Autodesk Inventor part; units mm, degrees
(part 2 of 2)
sketch "Sketch4" plane through (-0.0003, -144.9621, 0) normal (0, -1, 0) x (-0.0016, 0, -1)
  line L0 (16.9376, 64.7399) -> (58.7136, 64.7399) construction
  line L1 (58.7136, 64.7399) -> (58.7136, 48.1903) construction
  line L2 (58.7136, 48.1903) -> (16.9376, 48.1903) construction
  line L3 (16.9376, 48.1903) -> (16.9376, 64.7399) construction
  line L4 (19.529, 58.6329) -> (17.2049, 58.6329)
  line L5 (17.2049, 58.6329) -> (17.2049, 59.2456)
  line L6 (17.2049, 59.2456) -> (17.9682, 59.2456)
  line L7 (17.9682, 59.2456) -> (17.9682, 64.0203)
  line L8 (17.9682, 64.0203) -> (17.2049, 64.0203)
  line L9 (17.2049, 64.0203) -> (17.2049, 64.6329)
  line L10 (17.2049, 64.6329) -> (19.529, 64.6329)
  line L11 (19.529, 64.6329) -> (19.529, 64.0203)
  line L12 (19.529, 64.0203) -> (18.7656, 64.0203)
  line L13 (18.7656, 64.0203) -> (18.7656, 59.2456)
  line L14 (18.7656, 59.2456) -> (19.529, 59.2456)
  line L15 (19.529, 59.2456) -> (19.529, 58.6329)
  line L16 (24.8094, 58.6329) -> (23.9148, 58.6329)
  line L17 (23.9148, 58.6329) -> (21.26, 63.8063)
  line L18 (21.26, 63.8063) -> (21.26, 58.6329)
  line L19 (21.26, 58.6329) -> (20.5161, 58.6329)
  line L20 (20.5161, 58.6329) -> (20.5161, 64.6329)
  line L21 (20.5161, 64.6329) -> (21.649, 64.6329)
  line L22 (21.649, 64.6329) -> (24.0655, 59.8825)
  line L23 (24.0655, 59.8825) -> (24.0655, 64.6329)
  line L24 (24.0655, 64.6329) -> (24.8094, 64.6329)
  line L25 (24.8094, 64.6329) -> (24.8094, 58.6329)
  line L26 (27.4253, 58.6329) -> (27.4253, 63.923)
  line L27 (27.4253, 63.923) -> (25.4123, 63.923)
  line L28 (25.4123, 63.923) -> (25.4123, 64.6329)
  line L29 (25.4123, 64.6329) -> (30.2357, 64.6329)
  line L30 (30.2357, 64.6329) -> (30.2357, 63.923)
  line L31 (30.2357, 63.923) -> (28.2227, 63.923)
  line L32 (28.2227, 63.923) -> (28.2227, 58.6329)
  line L33 (28.2227, 58.6329) -> (27.4253, 58.6329)
  line L34 (30.8434, 58.6329) -> (30.8434, 64.6329)
  line L35 (30.8434, 64.6329) -> (34.5971, 64.6329)
  line L36 (34.5971, 64.6329) -> (34.5971, 63.923)
  line L37 (34.5971, 63.923) -> (31.6409, 63.923)
  line L38 (31.6409, 63.923) -> (31.6409, 62.2796)
  line L39 (31.6409, 62.2796) -> (34.3977, 62.2796)
  line L40 (34.3977, 62.2796) -> (34.3977, 61.5697)
  line L41 (34.3977, 61.5697) -> (31.6409, 61.5697)
  line L42 (31.6409, 61.5697) -> (31.6409, 59.3428)
  line L43 (31.6409, 59.3428) -> (34.5971, 59.3428)
  line L44 (34.5971, 59.3428) -> (34.5971, 58.6329)
  line L45 (34.5971, 58.6329) -> (30.8434, 58.6329)
  line L46 (40.1157, 58.6329) -> (39.0801, 58.6329)
  line L47 (39.0801, 58.6329) -> (37.1838, 61.0203)
  line L48 (37.1838, 61.0203) -> (36.2697, 61.0203)
  line L49 (36.2697, 61.0203) -> (36.2697, 58.6329)
  line L50 (36.2697, 58.6329) -> (35.4723, 58.6329)
  line L51 (35.4723, 58.6329) -> (35.4723, 64.6329)
  line L52 (35.4723, 64.6329) -> (37.0185, 64.6329)
  spline S0 degree 2 poles (37.0185, 64.6329) (37.5339, 64.6329) (38.2292, 64.5211) (38.5452, 64.3169) knots 0 0 0 1 2 2 2
  spline S1 degree 2 poles (38.5452, 64.3169) (38.8613, 64.1127) (39.2259, 63.4757) (39.2259, 63.0041) knots 0 0 0 1 2 2 2
  spline S2 degree 2 poles (39.2259, 63.0041) (39.2259, 62.3477) (38.555, 61.4579) (37.9812, 61.2439) knots 0 0 0 1 2 2 2
  line L53 (37.9812, 61.2439) -> (40.1157, 58.6329)
  spline S3 degree 2 poles (38.3945, 62.9409) (38.3945, 63.2034) (38.2097, 63.607) (38.0152, 63.7383) knots 0 0 0 1 2 2 2
  spline S4 degree 2 poles (38.0152, 63.7383) (37.8451, 63.8501) (37.3929, 63.9425) (37.0622, 63.9425) knots 0 0 0 1 2 2 2
  line L54 (37.0622, 63.9425) -> (36.2697, 63.9425)
  line L55 (36.2697, 63.9425) -> (36.2697, 61.6864)
  line L56 (36.2697, 61.6864) -> (36.9699, 61.6864)
  spline S5 degree 2 poles (36.9699, 61.6864) (37.3151, 61.6864) (37.8645, 61.808) (38.0541, 61.9976) knots 0 0 0 1 2 2 2
  spline S6 degree 2 poles (38.0541, 61.9976) (38.2292, 62.1629) (38.3945, 62.6297) (38.3945, 62.9409) knots 0 0 0 1 2 2 2
  line L57 (44.1806, 63.923) -> (41.3896, 63.923)
  line L58 (41.3896, 63.923) -> (41.3896, 62.231)
  line L59 (41.3896, 62.231) -> (44.0639, 62.231)
  line L60 (44.0639, 62.231) -> (44.0639, 61.5211)
  line L61 (44.0639, 61.5211) -> (41.3896, 61.5211)
  line L62 (41.3896, 61.5211) -> (41.3896, 58.6329)
  line L63 (41.3896, 58.6329) -> (40.5922, 58.6329)
  line L64 (40.5922, 58.6329) -> (40.5922, 64.6329)
  line L65 (40.5922, 64.6329) -> (44.1806, 64.6329)
  line L66 (44.1806, 64.6329) -> (44.1806, 63.923)
  line L67 (44.2486, 58.6329) -> (46.2713, 64.6329)
  line L68 (46.2713, 64.6329) -> (47.2535, 64.6329)
  line L69 (47.2535, 64.6329) -> (49.2762, 58.6329)
  line L70 (49.2762, 58.6329) -> (48.435, 58.6329)
  line L71 (48.435, 58.6329) -> (47.8904, 60.3104)
  line L72 (47.8904, 60.3104) -> (45.6003, 60.3104)
  line L73 (45.6003, 60.3104) -> (45.0558, 58.6329)
  line L74 (45.0558, 58.6329) -> (44.2486, 58.6329)
  line L75 (47.6716, 60.9911) -> (46.743, 63.8161)
  line L76 (46.743, 63.8161) -> (45.8191, 60.9911)
  line L77 (45.8191, 60.9911) -> (47.6716, 60.9911)
  spline S7 degree 2 poles (52.1887, 58.5259) (51.6052, 58.5259) (50.6182, 58.9198) (50.2584, 59.3136) knots 0 0 0 1 2 2 2
  spline S8 degree 2 poles (50.2584, 59.3136) (49.8986, 59.7026) (49.5047, 60.8695) (49.5047, 61.6281) knots 0 0 0 1 2 2 2
  spline S9 degree 2 poles (49.5047, 61.6281) (49.5047, 62.3817) (49.8888, 63.5) (50.2535, 63.9133) knots 0 0 0 1 2 2 2
  spline S10 degree 2 poles (50.2535, 63.9133) (50.6133, 64.3169) (51.5955, 64.7399) (52.2033, 64.7399) knots 0 0 0 1 2 2 2
  spline S11 degree 2 poles (52.2033, 64.7399) (52.5047, 64.7399) (53.0347, 64.6524) (53.2584, 64.5843) knots 0 0 0 1 2 2 2
  spline S12 degree 2 poles (53.2584, 64.5843) (53.4528, 64.5211) (53.8564, 64.3412) (54.0558, 64.2342) knots 0 0 0 1 2 2 2
  line L78 (54.0558, 64.2342) -> (54.0558, 63.2715)
  line L79 (54.0558, 63.2715) -> (53.9926, 63.2715)
  spline S13 degree 2 poles (53.9926, 63.2715) (53.8856, 63.3687) (53.555, 63.641) (53.3167, 63.7723) knots 0 0 0 1 2 2 2
  spline S14 degree 2 poles (53.3167, 63.7723) (53.0882, 63.8987) (52.5485, 64.0592) (52.1984, 64.0592) knots 0 0 0 1 2 2 2
  spline S15 degree 2 poles (52.1984, 64.0592) (51.8143, 64.0592) (51.1287, 63.7431) (50.871, 63.4417) knots 0 0 0 1 2 2 2
  spline S16 degree 2 poles (50.871, 63.4417) (50.6182, 63.1353) (50.3362, 62.2067) (50.3362, 61.6281) knots 0 0 0 1 2 2 2
  spline S17 degree 2 poles (50.3362, 61.6281) (50.3362, 61.0106) (50.6327, 60.1208) (50.8904, 59.8144) knots 0 0 0 1 2 2 2
  spline S18 degree 2 poles (50.8904, 59.8144) (51.1433, 59.5178) (51.8191, 59.2164) (52.1984, 59.2164) knots 0 0 0 1 2 2 2
  spline S19 degree 2 poles (52.1984, 59.2164) (52.5436, 59.2164) (53.1319, 59.3866) (53.3605, 59.513) knots 0 0 0 1 2 2 2
  spline S20 degree 2 poles (53.3605, 59.513) (53.5793, 59.6394) (53.905, 59.902) (53.9974, 59.9943) knots 0 0 0 1 2 2 2
  line L80 (53.9974, 59.9943) -> (54.0558, 59.9943)
  line L81 (54.0558, 59.9943) -> (54.0558, 59.0413)
  spline S21 degree 2 poles (54.0558, 59.0413) (53.8564, 58.949) (53.5063, 58.7788) (53.2584, 58.701) knots 0 0 0 1 2 2 2
  spline S22 degree 2 poles (53.2584, 58.701) (52.9958, 58.6135) (52.5485, 58.5259) (52.1887, 58.5259) knots 0 0 0 1 2 2 2
  line L82 (54.7997, 58.6329) -> (54.7997, 64.6329)
  line L83 (54.7997, 64.6329) -> (58.5533, 64.6329)
  line L84 (58.5533, 64.6329) -> (58.5533, 63.923)
  line L85 (58.5533, 63.923) -> (55.5971, 63.923)
  line L86 (55.5971, 63.923) -> (55.5971, 62.2796)
  line L87 (55.5971, 62.2796) -> (58.354, 62.2796)
  line L88 (58.354, 62.2796) -> (58.354, 61.5697)
  line L89 (58.354, 61.5697) -> (55.5971, 61.5697)
  line L90 (55.5971, 61.5697) -> (55.5971, 59.3428)
  line L91 (55.5971, 59.3428) -> (58.5533, 59.3428)
  line L92 (58.5533, 59.3428) -> (58.5533, 58.6329)
  line L93 (58.5533, 58.6329) -> (54.7997, 58.6329)
  line L94 (27.6076, 48.7541) -> (26.8102, 48.7541)
  line L95 (26.8102, 48.7541) -> (26.8102, 53.9226)
  line L96 (26.8102, 53.9226) -> (25.2446, 50.4072)
  line L97 (25.2446, 50.4072) -> (24.7584, 50.4072)
  line L98 (24.7584, 50.4072) -> (23.2073, 53.9226)
  line L99 (23.2073, 53.9226) -> (23.2073, 48.7541)
  line L100 (23.2073, 48.7541) -> (22.4634, 48.7541)
  line L101 (22.4634, 48.7541) -> (22.4634, 54.7541)
  line L102 (22.4634, 54.7541) -> (23.5525, 54.7541)
  line L103 (23.5525, 54.7541) -> (25.0501, 51.4137)
  line L104 (25.0501, 51.4137) -> (26.499, 54.7541)
  line L105 (26.499, 54.7541) -> (27.6076, 54.7541)
  line L106 (27.6076, 54.7541) -> (27.6076, 48.7541)
  spline S23 degree 2 poles (33.0679, 54.0685) (33.4083, 53.6698) (33.7875, 52.5029) (33.7875, 51.7541) knots 0 0 0 1 2 2 2
  spline S24 degree 2 poles (33.7875, 51.7541) (33.7875, 51.0247) (33.418, 49.8432) (33.0679, 49.4445) knots 0 0 0 1 2 2 2
  spline S25 degree 2 poles (33.0679, 49.4445) (32.6984, 49.0264) (31.7211, 48.6277) (31.1327, 48.6277) knots 0 0 0 1 2 2 2
  spline S26 degree 2 poles (31.1327, 48.6277) (30.525, 48.6277) (29.5525, 49.0409) (29.1976, 49.4445) knots 0 0 0 1 2 2 2
  spline S27 degree 2 poles (29.1976, 49.4445) (28.8524, 49.8432) (28.4828, 51.015) (28.4828, 51.7541) knots 0 0 0 1 2 2 2
  spline S28 degree 2 poles (28.4828, 51.7541) (28.4828, 52.5077) (28.8572, 53.6552) (29.2024, 54.0685) knots 0 0 0 1 2 2 2
  spline S29 degree 2 poles (29.2024, 54.0685) (29.5525, 54.4672) (30.5298, 54.8805) (31.1327, 54.8805) knots 0 0 0 1 2 2 2
  spline S30 degree 2 poles (31.1327, 54.8805) (31.7454, 54.8805) (32.7276, 54.4526) (33.0679, 54.0685) knots 0 0 0 1 2 2 2
  spline S31 degree 2 poles (32.9561, 51.7541) (32.9561, 52.3473) (32.6984, 53.2662) (32.465, 53.5677) knots 0 0 0 1 2 2 2
  spline S32 degree 2 poles (32.465, 53.5677) (32.2268, 53.8789) (31.5558, 54.1901) (31.1376, 54.1901) knots 0 0 0 1 2 2 2
  spline S33 degree 2 poles (31.1376, 54.1901) (30.7049, 54.1901) (30.0533, 53.8886) (29.8054, 53.5677) knots 0 0 0 1 2 2 2
  spline S34 degree 2 poles (29.8054, 53.5677) (29.5671, 53.2614) (29.3143, 52.3375) (29.3143, 51.7541) knots 0 0 0 1 2 2 2
  spline S35 degree 2 poles (29.3143, 51.7541) (29.3143, 50.5726) (30.3062, 49.3181) (31.1376, 49.3181) knots 0 0 0 1 2 2 2
  spline S36 degree 2 poles (31.1376, 49.3181) (31.9691, 49.3181) (32.9561, 50.5726) (32.9561, 51.7541) knots 0 0 0 1 2 2 2
  spline S37 degree 2 poles (39.3937, 51.7492) (39.3937, 50.9275) (38.7276, 49.605) (38.1684, 49.2354) knots 0 0 0 1 2 2 2
  spline S38 degree 2 poles (38.1684, 49.2354) (37.7114, 48.9486) (36.7729, 48.7541) (36.0436, 48.7541) knots 0 0 0 1 2 2 2
  line L107 (36.0436, 48.7541) -> (34.6627, 48.7541)
  line L108 (34.6627, 48.7541) -> (34.6627, 54.7541)
  line L109 (34.6627, 54.7541) -> (36.029, 54.7541)
  spline S39 degree 2 poles (36.029, 54.7541) (36.8751, 54.7541) (37.8378, 54.5012) (38.1781, 54.2776) knots 0 0 0 1 2 2 2
  spline S40 degree 2 poles (38.1781, 54.2776) (38.7567, 53.8935) (39.3937, 52.6244) (39.3937, 51.7492) knots 0 0 0 1 2 2 2
  spline S41 degree 2 poles (38.5622, 51.7589) (38.5622, 52.4494) (38.1052, 53.4267) (37.653, 53.7038) knots 0 0 0 1 2 2 2
  spline S42 degree 2 poles (37.653, 53.7038) (37.3321, 53.8935) (36.6076, 54.0636) (36.0679, 54.0636) knots 0 0 0 1 2 2 2
  line L110 (36.0679, 54.0636) -> (35.4601, 54.0636)
  line L111 (35.4601, 54.0636) -> (35.4601, 49.4445)
  line L112 (35.4601, 49.4445) -> (36.0679, 49.4445)
  spline S43 degree 2 poles (36.0679, 49.4445) (36.5979, 49.4445) (37.4002, 49.6147) (37.7259, 49.8432) knots 0 0 0 1 2 2 2
  spline S44 degree 2 poles (37.7259, 49.8432) (38.1441, 50.1252) (38.5622, 51.0588) (38.5622, 51.7589) knots 0 0 0 1 2 2 2
  spline S45 degree 2 poles (42.3548, 48.6277) (41.8248, 48.6277) (41.0371, 48.9048) (40.76, 49.182) knots 0 0 0 1 2 2 2
  spline S46 degree 2 poles (40.76, 49.182) (40.4439, 49.4931) (40.1862, 50.3683) (40.1862, 51.0102) knots 0 0 0 1 2 2 2
  line L113 (40.1862, 51.0102) -> (40.1862, 54.7541)
  line L114 (40.1862, 54.7541) -> (40.9836, 54.7541)
  line L115 (40.9836, 54.7541) -> (40.9836, 51.0102)
  spline S47 degree 2 poles (40.9836, 51.0102) (40.9836, 50.592) (41.0906, 50.028) (41.2413, 49.7995) knots 0 0 0 1 2 2 2
  spline S48 degree 2 poles (41.2413, 49.7995) (41.4018, 49.5563) (41.9561, 49.3084) (42.3548, 49.3084) knots 0 0 0 1 2 2 2
  spline S49 degree 2 poles (42.3548, 49.3084) (42.7292, 49.3084) (43.3127, 49.5563) (43.4731, 49.7995) knots 0 0 0 1 2 2 2
  spline S50 degree 2 poles (43.4731, 49.7995) (43.6238, 50.028) (43.7308, 50.5871) (43.7308, 50.9907) knots 0 0 0 1 2 2 2
  line L116 (43.7308, 50.9907) -> (43.7308, 54.7541)
  line L117 (43.7308, 54.7541) -> (44.5282, 54.7541)
  line L118 (44.5282, 54.7541) -> (44.5282, 51.0102)
  spline S51 degree 2 poles (44.5282, 51.0102) (44.5282, 50.3829) (44.2754, 49.4883) (43.9545, 49.182) knots 0 0 0 1 2 2 2
  spline S52 degree 2 poles (43.9545, 49.182) (43.6676, 48.8999) (42.9091, 48.6277) (42.3548, 48.6277) knots 0 0 0 1 2 2 2
  line L119 (49.1473, 48.7541) -> (45.6708, 48.7541)
  line L120 (45.6708, 48.7541) -> (45.6708, 54.7541)
  line L121 (45.6708, 54.7541) -> (46.4682, 54.7541)
  line L122 (46.4682, 54.7541) -> (46.4682, 49.464)
  line L123 (46.4682, 49.464) -> (49.1473, 49.464)
  line L124 (49.1473, 49.464) -> (49.1473, 48.7541)
  line L125 (49.7746, 48.7541) -> (49.7746, 54.7541)
  line L126 (49.7746, 54.7541) -> (53.5282, 54.7541)
  line L127 (53.5282, 54.7541) -> (53.5282, 54.0442)
  line L128 (53.5282, 54.0442) -> (50.572, 54.0442)
  line L129 (50.572, 54.0442) -> (50.572, 52.4008)
  line L130 (50.572, 52.4008) -> (53.3289, 52.4008)
  line L131 (53.3289, 52.4008) -> (53.3289, 51.6909)
  line L132 (53.3289, 51.6909) -> (50.572, 51.6909)
  line L133 (50.572, 51.6909) -> (50.572, 49.464)
  line L134 (50.572, 49.464) -> (53.5282, 49.464)
  line L135 (53.5282, 49.464) -> (53.5282, 48.7541)
  line L136 (53.5282, 48.7541) -> (49.7746, 48.7541)
  point P0 (0, 0)
  constraints: 2 other
extrude "Extrusion4" add sketch "Sketch4" against normal blind 2
ref_plane "Work Plane5" through (-0.0003, -144.9621, -142.4319) normal (0, 0, -1) x (-1, 0, 0)
sketch "Sketch5" plane through (-0.0003, -144.9621, -142.4319) normal (0, 0, -1) x (-1, 0, 0)
  circle A0 centre (-58.0001, 28.9999) radius 17.5
  circle A1 centre (-58.0002, 115.962) radius 17.5
  spline S0 degree 2 poles (-56.1337, 59.9308) (-56.1337, 60.7898) (-55.9473, 61.9487) (-55.6069, 62.4754) knots -2 -2 -2 -1 0 0 0 projected
  spline S1 degree 2 poles (-55.6069, 62.4754) (-55.2666, 63.0022) (-54.205, 63.6099) (-53.4189, 63.6099) knots -2 -2 -2 -1 0 0 0 projected
  spline S2 degree 2 poles (-53.4189, 63.6099) (-52.3249, 63.6099) (-50.8419, 62.4916) (-50.4854, 61.5354) knots -2 -2 -2 -1 0 0 0 projected
  line L0 (-50.4854, 61.5354) -> (-46.1337, 65.0929) projected
  line L1 (-46.1337, 65.0929) -> (-46.1337, 63.3668) projected
  line L2 (-46.1337, 63.3668) -> (-50.1126, 60.2064) projected
  line L3 (-50.1126, 60.2064) -> (-50.1126, 58.6829) projected
  line L4 (-50.1126, 58.6829) -> (-46.1337, 58.6829) projected
  line L5 (-46.1337, 58.6829) -> (-46.1337, 57.3539) projected
  line L6 (-46.1337, 57.3539) -> (-56.1337, 57.3539) projected
  line L7 (-56.1337, 57.3539) -> (-56.1337, 59.9308) projected
  spline S3 degree 2 poles (-35.1604, 55.2567) (-35.692, 54.7964) (-37.2544, 54.3037) (-38.2398, 54.3037) knots -2 -2 -2 -1 0 0 0 projected
  spline S4 degree 2 poles (-38.2398, 54.3037) (-39.2446, 54.3037) (-40.7746, 54.8028) (-41.3257, 55.2631) knots -2 -2 -2 -1 0 0 0 projected
  spline S5 degree 2 poles (-41.3257, 55.2631) (-41.8573, 55.7299) (-42.4083, 57.033) (-42.4083, 57.8369) knots -2 -2 -2 -1 0 0 0 projected
  spline S6 degree 2 poles (-42.4083, 57.8369) (-42.4083, 58.6537) (-41.8378, 59.9633) (-41.3257, 60.4171) knots -2 -2 -2 -1 0 0 0 projected
  spline S7 degree 2 poles (-41.3257, 60.4171) (-40.7941, 60.8709) (-39.2382, 61.3766) (-38.2398, 61.3766) knots -2 -2 -2 -1 0 0 0 projected
  spline S8 degree 2 poles (-38.2398, 61.3766) (-37.2673, 61.3766) (-35.692, 60.8839) (-35.1604, 60.4171) knots -2 -2 -2 -1 0 0 0 projected
  spline S9 degree 2 poles (-35.1604, 60.4171) (-34.6028, 59.9244) (-34.0712, 58.6213) (-34.0712, 57.8369) knots -2 -2 -2 -1 0 0 0 projected
  spline S10 degree 2 poles (-34.0712, 57.8369) (-34.0712, 57.0265) (-34.6223, 55.7299) (-35.1604, 55.2567) knots -2 -2 -2 -1 0 0 0 projected
  line L8 (-38.1555, 82.7186) -> (-35.1863, 82.7186) projected
  line L9 (-35.1863, 82.7186) -> (-35.1863, 86.6602) projected
  line L10 (-35.1863, 86.6602) -> (-34.2398, 86.6602) projected
  line L11 (-34.2398, 86.6602) -> (-34.2398, 81.6554) projected
  line L12 (-34.2398, 81.6554) -> (-42.2398, 81.6554) projected
  line L13 (-42.2398, 81.6554) -> (-42.2398, 86.6602) projected
  line L14 (-42.2398, 86.6602) -> (-41.2933, 86.6602) projected
  line L15 (-41.2933, 86.6602) -> (-41.2933, 82.7186) projected
  line L16 (-41.2933, 82.7186) -> (-39.102, 82.7186) projected
  line L17 (-39.102, 82.7186) -> (-39.102, 86.3944) projected
  line L18 (-39.102, 86.3944) -> (-38.1555, 86.3944) projected
  line L19 (-38.1555, 86.3944) -> (-38.1555, 82.7186) projected
  line L20 (-42.2398, 76.1837) -> (-42.2398, 77.2469) projected
  line L21 (-42.2398, 77.2469) -> (-35.1863, 77.2469) projected
  line L22 (-35.1863, 77.2469) -> (-35.1863, 80.8191) projected
  line L23 (-35.1863, 80.8191) -> (-34.2398, 80.8191) projected
  line L24 (-34.2398, 80.8191) -> (-34.2398, 76.1837) projected
  line L25 (-34.2398, 76.1837) -> (-42.2398, 76.1837) projected
  line L26 (-16.862, 12.0764) -> (-28.862, 12.0764) projected
  line L27 (-28.862, 12.0764) -> (-28.862, 15.091) projected
  spline S11 degree 2 poles (-28.862, 15.091) (-28.862, 16.1607) (-28.5119, 17.6583) (-28.1132, 18.232) knots -2 -2 -2 -1 0 0 0 projected
  spline S12 degree 2 poles (-28.1132, 18.232) (-27.6561, 18.903) (-26.2461, 19.6615) (-25.2445, 19.6615) knots -2 -2 -2 -1 0 0 0 projected
  spline S13 degree 2 poles (-25.2445, 19.6615) (-24.4665, 19.6615) (-23.0662, 19.1072) (-22.58, 18.6113) knots -2 -2 -2 -1 0 0 0 projected
  spline S14 degree 2 poles (-22.58, 18.6113) (-21.9673, 17.9889) (-21.3352, 16.3066) (-21.3352, 15.0229) knots -2 -2 -2 -1 0 0 0 projected
  line L28 (-21.3352, 15.0229) -> (-21.3352, 13.6712) projected
  line L29 (-21.3352, 13.6712) -> (-16.862, 13.6712) projected
  line L30 (-16.862, 13.6712) -> (-16.862, 12.0764) projected
  line L31 (-10.1757, 135.4385) -> (-10.1757, 136.2683) projected
  line L32 (-10.1757, 136.2683) -> (-2.9666, 136.2683) projected
  line L33 (-2.9666, 136.2683) -> (-2.9666, 137.688) projected
  line L34 (-2.9666, 137.688) -> (-2.1497, 137.688) projected
  line L35 (-2.1497, 137.688) -> (-2.1497, 133.7853) projected
  line L36 (-2.1497, 133.7853) -> (-2.9666, 133.7853) projected
  line L37 (-2.9666, 133.7853) -> (-2.9666, 135.2375) projected
  line L38 (-2.9666, 135.2375) -> (-8.328, 135.2375) projected
  line L39 (-8.328, 135.2375) -> (-8.328, 133.7853) projected
  line L40 (-8.328, 133.7853) -> (-9.0606, 133.7853) projected
  spline S15 degree 2 poles (-9.0606, 133.7853) (-9.0606, 134.6086) (-9.5274, 135.3866) (-10.1757, 135.4385) knots -2 -2 -2 -1 0 0 0 projected
  line L41 (-46.0033, 83.678) -> (-46.0033, 82.349) projected
  line L42 (-46.0033, 82.349) -> (-56.0033, 82.349) projected
  line L43 (-56.0033, 82.349) -> (-56.0033, 88.3295) projected
  line L44 (-56.0033, 88.3295) -> (-54.8201, 88.3295) projected
  line L45 (-54.8201, 88.3295) -> (-54.8201, 83.678) projected
  line L46 (-54.8201, 83.678) -> (-52, 83.678) projected
  line L47 (-52, 83.678) -> (-52, 88.135) projected
  line L48 (-52, 88.135) -> (-50.8169, 88.135) projected
  line L49 (-50.8169, 88.135) -> (-50.8169, 83.678) projected
  line L50 (-50.8169, 83.678) -> (-46.0033, 83.678) projected
  line L51 (-42.2398, 67.1724) -> (-42.2398, 68.2356) projected
  line L52 (-42.2398, 68.2356) -> (-37.2479, 68.2356) projected
  spline S16 degree 2 poles (-37.2479, 68.2356) (-36.4116, 68.2356) (-35.2187, 67.8985) (-34.8103, 67.4706) knots -2 -2 -2 -1 0 0 0 projected
  spline S17 degree 2 poles (-34.8103, 67.4706) (-34.4343, 67.0881) (-34.0712, 66.0768) (-34.0712, 65.3377) knots -2 -2 -2 -1 0 0 0 projected
  spline S18 degree 2 poles (-34.0712, 65.3377) (-34.0712, 64.631) (-34.4408, 63.5808) (-34.8103, 63.2113) knots -2 -2 -2 -1 0 0 0 projected
  spline S19 degree 2 poles (-34.8103, 63.2113) (-35.2252, 62.7899) (-36.3921, 62.4463) (-37.2479, 62.4463) knots -2 -2 -2 -1 0 0 0 projected
  line L53 (-37.2479, 62.4463) -> (-42.2398, 62.4463) projected
  line L54 (-42.2398, 62.4463) -> (-42.2398, 63.5095) projected
  line L55 (-42.2398, 63.5095) -> (-37.2479, 63.5095) projected
  spline S20 degree 2 poles (-37.2479, 63.5095) (-36.6904, 63.5095) (-35.9383, 63.6521) (-35.6336, 63.8531) knots -2 -2 -2 -1 0 0 0 projected
  spline S21 degree 2 poles (-35.6336, 63.8531) (-35.3095, 64.067) (-34.9788, 64.8061) (-34.9788, 65.3377) knots -2 -2 -2 -1 0 0 0 projected
  spline S22 degree 2 poles (-34.9788, 65.3377) (-34.9788, 65.8369) (-35.3095, 66.6148) (-35.6336, 66.8288) knots -2 -2 -2 -1 0 0 0 projected
  spline S23 degree 2 poles (-35.6336, 66.8288) (-35.9383, 67.0298) (-36.6839, 67.1724) (-37.222, 67.1724) knots -2 -2 -2 -1 0 0 0 projected
  line L56 (-37.222, 67.1724) -> (-42.2398, 67.1724) projected
  line L57 (-42.2398, 93.4414) -> (-41.2933, 93.4414) projected
  line L58 (-41.2933, 93.4414) -> (-41.2933, 90.7575) projected
  line L59 (-41.2933, 90.7575) -> (-34.2398, 90.7575) projected
  line L60 (-34.2398, 90.7575) -> (-34.2398, 89.6943) projected
  line L61 (-34.2398, 89.6943) -> (-41.2933, 89.6943) projected
  line L62 (-41.2933, 89.6943) -> (-41.2933, 87.0103) projected
  line L63 (-41.2933, 87.0103) -> (-42.2398, 87.0103) projected
  line L64 (-42.2398, 87.0103) -> (-42.2398, 93.4414) projected
  line L65 (-42.2398, 75.3733) -> (-41.2933, 75.3733) projected
  line L66 (-41.2933, 75.3733) -> (-41.2933, 72.6894) projected
  line L67 (-41.2933, 72.6894) -> (-34.2398, 72.6894) projected
  line L68 (-34.2398, 72.6894) -> (-34.2398, 71.6262) projected
  line L69 (-34.2398, 71.6262) -> (-41.2933, 71.6262) projected
  line L70 (-41.2933, 71.6262) -> (-41.2933, 68.9422) projected
  line L71 (-41.2933, 68.9422) -> (-42.2398, 68.9422) projected
  line L72 (-42.2398, 68.9422) -> (-42.2398, 75.3733) projected
  line L73 (-19.5848, 29.4832) -> (-19.5848, 29.5999) projected
  line L74 (-19.5848, 29.5999) -> (-17.6788, 29.5999) projected
  spline S24 degree 2 poles (-17.6788, 29.5999) (-17.4941, 29.2012) (-17.1537, 28.501) (-16.9981, 28.0051) knots -2 -2 -2 -1 0 0 0 projected
  spline S25 degree 2 poles (-16.9981, 28.0051) (-16.8231, 27.48) (-16.648, 26.5853) (-16.648, 25.8657) knots -2 -2 -2 -1 0 0 0 projected
  spline S26 degree 2 poles (-16.648, 25.8657) (-16.648, 24.6988) (-17.4357, 22.7247) (-18.2234, 22.0051) knots -2 -2 -2 -1 0 0 0 projected
  spline S27 degree 2 poles (-18.2234, 22.0051) (-19.0014, 21.2855) (-21.3352, 20.4978) (-22.8523, 20.4978) knots -2 -2 -2 -1 0 0 0 projected
  spline S28 degree 2 poles (-22.8523, 20.4978) (-24.3596, 20.4978) (-26.5962, 21.266) (-27.4228, 21.9954) knots -2 -2 -2 -1 0 0 0 projected
  spline S29 degree 2 poles (-27.4228, 21.9954) (-28.2299, 22.715) (-29.0759, 24.6793) (-29.0759, 25.8949) knots -2 -2 -2 -1 0 0 0 projected
  spline S30 degree 2 poles (-29.0759, 25.8949) (-29.0759, 26.4978) (-28.9009, 27.5578) (-28.7647, 28.0051) knots -2 -2 -2 -1 0 0 0 projected
  spline S31 degree 2 poles (-28.7647, 28.0051) (-28.6383, 28.3941) (-28.2785, 29.2012) (-28.0646, 29.5999) knots -2 -2 -2 -1 0 0 0 projected
  line L75 (-28.0646, 29.5999) -> (-26.1391, 29.5999) projected
  line L76 (-26.1391, 29.5999) -> (-26.1391, 29.4735) projected
  spline S32 degree 2 poles (-26.1391, 29.4735) (-26.3336, 29.2596) (-26.8782, 28.5983) (-27.1408, 28.1218) knots -2 -2 -2 -1 0 0 0 projected
  spline S33 degree 2 poles (-27.1408, 28.1218) (-27.3936, 27.6647) (-27.7145, 26.5853) (-27.7145, 25.8852) knots -2 -2 -2 -1 0 0 0 projected
  spline S34 degree 2 poles (-27.7145, 25.8852) (-27.7145, 25.1169) (-27.0824, 23.7458) (-26.4795, 23.2304) knots -2 -2 -2 -1 0 0 0 projected
  spline S35 degree 2 poles (-26.4795, 23.2304) (-25.8668, 22.7247) (-24.0095, 22.1607) (-22.8523, 22.1607) knots -2 -2 -2 -1 0 0 0 projected
  spline S36 degree 2 poles (-22.8523, 22.1607) (-21.6173, 22.1607) (-19.8377, 22.7539) (-19.225, 23.2693) knots -2 -2 -2 -1 0 0 0 projected
  spline S37 degree 2 poles (-19.225, 23.2693) (-18.6318, 23.775) (-18.0289, 25.1267) (-18.0289, 25.8852) knots -2 -2 -2 -1 0 0 0 projected
  spline S38 degree 2 poles (-18.0289, 25.8852) (-18.0289, 26.5756) (-18.3693, 27.7523) (-18.6221, 28.2093) knots -2 -2 -2 -1 0 0 0 projected
  spline S39 degree 2 poles (-18.6221, 28.2093) (-18.8749, 28.6469) (-19.4001, 29.2985) (-19.5848, 29.4832) knots -2 -2 -2 -1 0 0 0 projected
  spline S40 degree 2 poles (-10.1497, 128.6184) (-10.1497, 129.3056) (-10.0006, 130.2326) (-9.7283, 130.654) knots -2 -2 -2 -1 0 0 0 projected
  spline S41 degree 2 poles (-9.7283, 130.654) (-9.4561, 131.0754) (-8.6068, 131.5616) (-7.9779, 131.5616) knots -2 -2 -2 -1 0 0 0 projected
  spline S42 degree 2 poles (-7.9779, 131.5616) (-7.1027, 131.5616) (-5.9163, 130.667) (-5.6311, 129.902) knots -2 -2 -2 -1 0 0 0 projected
  line L77 (-5.6311, 129.902) -> (-2.1497, 132.748) projected
  line L78 (-2.1497, 132.748) -> (-2.1497, 131.3671) projected
  line L79 (-2.1497, 131.3671) -> (-5.3329, 128.8388) projected
  line L80 (-5.3329, 128.8388) -> (-5.3329, 127.62) projected
  line L81 (-5.3329, 127.62) -> (-2.1497, 127.62) projected
  line L82 (-2.1497, 127.62) -> (-2.1497, 126.5568) projected
  line L83 (-2.1497, 126.5568) -> (-10.1497, 126.5568) projected
  line L84 (-10.1497, 126.5568) -> (-10.1497, 128.6184) projected
  line L85 (3, 2) -> (-80, 1.9999) projected
  line L86 (2.9997, 142.9621) -> (3, 2) projected
  line L87 (-80.0003, 142.9619) -> (2.9997, 142.9621) projected
  line L88 (-80, 1.9999) -> (-80.0003, 142.9619) projected
  circle A2 centre (-65.2412, 59.9999) radius 3.35 projected
  circle A3 centre (-65.2412, 84.962) radius 3.35 projected
  line L89 (-4.0356, 12.0349) -> (-14.0356, 12.0349) projected
  line L90 (-14.0356, 12.0349) -> (-14.0357, 29.0349) projected
  line L91 (-14.0357, 29.0349) -> (-4.0357, 29.0349) projected
  line L92 (-4.0357, 29.0349) -> (-4.0356, 12.0349) projected
  circle A4 centre (-58.0001, 28.9999) radius 15
  circle A5 centre (-58.0002, 115.962) radius 15
  circle A6 centre (-58.0001, 28.9999) radius 17.5 projected
  circle A7 centre (-58.0002, 115.962) radius 17.5 projected
  point P0 (-0.0003, 144.9621)
  dimension "d8" = 35
  dimension "d9" = 35
  dimension "d10" = 22
  dimension "d11" = 27
  dimension "d12" = 27
  dimension "d13" = 22
  dimension "d14" = 30
  dimension "d15" = 30
  constraints: 4 centre point, 2 coincident
  measures "d8" diameter of A0
  measures "d9" diameter of A1
  measures "d10" distance from line of A1.centre L88
  measures "d11" distance from line of L87 A1.centre
  measures "d12" distance from line of L85 A0.centre
  measures "d13" distance from line of L88 A0.centre
  measures "d14" diameter of A4
  measures "d15" diameter of A5
extrude "Extrusion5" add sketch "Sketch5" against normal blind 2 contours A0 | A1
body "Solid1"
